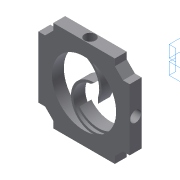
# Autodesk Inventor part: 50_Cube_Insert_Thorlabs
Saved by Autodesk Inventor 2019 (Build 230136000, 136)
## iProperties
Created: 2019-07-01
Part Number: 50_Cube_Insert_Thorlabs
Material: Generic
Document SubType Name: Modeling
Designer: diederichbenedict
Density: 1 g/cm^3
Appearance: Default
Author: diederichbenedict
Autodesk Inventor part; units mm, degrees
ref_plane "YZ Plane" through (0, 0, 0) normal (1, 0, 0) x (0, 1, 0)
ref_plane "Work Plane1" through (0, 0, 10) normal (0, 0, 1) x (1, 0, 0)
sketch "Sketch1" plane through (0, 0, 10) normal (0, 0, 1) x (1, 0, 0)
  line L0 (-4.0299, -0.3538) -> (-2.2322, 1.4439) construction
  arc A0 (-1.4439, 2.2322) -> (-2.2322, 1.4439) centre (-0.9299, 0.9299) ccw construction
  line L1 (-1.4439, 2.2322) -> (0.3538, 4.0299) construction
  line L2 (-37.8299, 42.2137) -> (-37.8299, 45.8299) construction
  line L3 (-37.8299, 45.8299) -> (-4.0299, 45.8299) construction
  line L4 (-4.0299, 45.8299) -> (-4.0299, 42.2137) construction
  line L5 (-4.0299, 4.0299) -> (0.3538, 4.0299) projected
  line L6 (-20.9299, 58.9723) -> (17.1124, 20.9299) construction
  line L7 (17.1124, 20.9299) -> (-20.9299, -17.1124) construction
  line L8 (-20.9299, -17.1124) -> (-58.9723, 20.9299) construction
  line L9 (-58.9723, 20.9299) -> (-20.9299, 58.9723) construction
  line L10 (-20.9299, 58.9723) -> (-20.9299, -17.1124) construction
  line L11 (17.1124, 20.9299) -> (-58.9723, 20.9299) construction
  line L12 (-20.9299, 58.9723) -> (32.8701, 58.9723) construction
  line L13 (-43.4299, 43.4299) -> (1.5701, 43.4299) construction
  line L14 (1.5701, 43.4299) -> (1.5701, -1.5701) construction
  line L15 (1.5701, -1.5701) -> (-43.4299, -1.5701) construction
  line L16 (-43.4299, -1.5701) -> (-43.4299, 43.4299) construction
  line L17 (-43.4299, 43.4299) -> (1.5701, -1.5701) construction
  line L18 (1.5701, 43.4299) -> (-43.4299, -1.5701) construction
  line L19 (-43.4299, 5.3876) -> (-43.4299, 36.4723)
  line L20 (-43.4299, 36.4723) -> (-36.4723, 43.4299)
  line L21 (-36.4723, 43.4299) -> (-5.3876, 43.4299)
  line L22 (-5.3876, 43.4299) -> (1.5701, 36.4723)
  line L23 (1.5701, 36.4723) -> (1.5701, 5.3876)
  line L24 (1.5701, 5.3876) -> (-5.3876, -1.5701)
  line L25 (-5.3876, -1.5701) -> (-36.4723, -1.5701)
  line L26 (-36.4723, -1.5701) -> (-43.4299, 5.3876)
  line L27 (-4.0299, 42.2137) -> (-37.8299, 42.2137) projected
  line L28 (-4.0299, -0.3538) -> (-4.0299, 4.0299) projected
  circle A1 centre (-20.9299, 20.9299) radius 13.3985
  circle A2 centre (-20.9299, 20.9299) radius 15.4895
  point P0 (-37.8299, 4.0299)
  dimension "d18" = 53.8
  dimension "d19" = 45
  dimension "d20" = 53.8
  dimension "d21" = 45
  dimension "d22" = 45
  dimension "d30" = 26.797
  dimension "d36" = 30.979
  constraints: 42 end point, 15 point on line, 4 parallel, 3 midpoint, 3 perpendicular, 2 centre point, 2 coincident, 2 horizontal, 1 equal length
  measures "d18" distance of L6.start L6.end
  measures "d19" angle of L6 L12
  measures "d20" distance of L6.end L7.end
  measures "d21" distance of L14.end L15.end
  measures "d22" distance of L13.end L14.end
  measures "d30" diameter of A1
  measures "d36" diameter of A2
extrude "Extrusion1" add sketch "Sketch1" along normal blind 6.5 contours L28 L24 L25 L26 L19 L20 L27 L22 L23 L5 | L5 L24 L28 | L27 L20 L21 L22 | A1 | A2
ref_plane "Work Plane2" through (-40.9959, 0.8639, 22.2359) normal (0, 0, 1) x (1, 0, 0)
sketch "Sketch3" plane through (0, 0, 10) normal (0, 0, -1) x (-1, 0, 0)
  line L0 (37.8299, -0.4701) -> (37.8299, 4.0299) construction
  line L1 (4.0299, 4.0299) -> (4.0299, -0.4701) construction
  line L2 (37.8299, -0.4701) -> (37.8299, 1.1886) construction
  line L3 (4.0299, -3.9701) -> (4.0299, -0.3538) construction
  line L4 (45.8299, 4.0299) -> (42.2137, 4.0299) construction
  line L5 (-0.3538, 4.0299) -> (-3.9701, 4.0299) construction
  line L6 (-3.9701, 37.8299) -> (-0.3538, 37.8299) construction
  line L7 (4.0299, 42.2137) -> (4.0299, 45.8299) construction
  line L8 (37.8299, 45.8299) -> (37.8299, 42.2137) construction
  line L9 (42.2137, 37.8299) -> (45.8299, 37.8299) construction
  line L10 (37.8299, 37.7299) -> (45.8299, 37.7299)
  line L11 (45.8299, 37.7299) -> (45.8299, 4.1299)
  line L12 (45.8299, 4.1299) -> (37.8299, 4.1299)
  line L13 (37.8299, 4.1299) -> (37.8299, 37.7299)
  line L14 (37.7299, 4.0299) -> (4.1299, 4.0299)
  line L15 (4.1299, 4.0299) -> (4.1299, -3.9701)
  line L16 (4.1299, -3.9701) -> (37.7299, -3.9701)
  line L17 (37.7299, -3.9701) -> (37.7299, 4.0299)
  line L18 (4.0299, 4.1299) -> (-3.9701, 4.1299)
  line L19 (-3.9701, 4.1299) -> (-3.9701, 37.7299)
  line L20 (-3.9701, 37.7299) -> (4.0299, 37.7299)
  line L21 (4.0299, 37.7299) -> (4.0299, 4.1299)
  line L22 (4.1299, 37.8299) -> (37.7299, 37.8299)
  line L23 (37.7299, 37.8299) -> (37.7299, 45.8299)
  line L24 (37.7299, 45.8299) -> (4.1299, 45.8299)
  line L25 (4.1299, 45.8299) -> (4.1299, 37.8299)
  point P0 (0, 0)
  dimension "d23" = 0.1
  dimension "d24" = 0.1
  dimension "d25" = 0.1
  dimension "d26" = 0.1
  dimension "d27" = 0.1
  constraints: 32 end point, 8 parallel, 4 horizontal, 4 perpendicular, 3 point on line
  measures "d23" distance between parallel lines of L8 L23
  measures "d24" distance between parallel lines of L7 L25
  measures "d25" distance between parallel lines of L6 L20
  measures "d26" distance between parallel lines of L5 L18
  measures "d27" distance between parallel lines of L1 L15
extrude "Extrusion3" add sketch "Sketch3" against normal up to surface (6.5 mm away)
sketch "Sketch6" plane through (0, 0, 16.5) normal (0, 0, 1) x (1, 0, 0)
  circle A0 centre (-20.9299, 20.9299) radius 17.5
  circle A1 centre (-20.9299, 20.9299) radius 13.3985
  line L0 (-45.8299, 4.1299) -> (-45.8299, 37.7299) projected
  line L1 (-4.1299, -3.9701) -> (-37.7299, -3.9701) projected
  line L2 (-37.7299, 45.8299) -> (-4.1299, 45.8299) projected
  point P0 (0, 0)
  point P1 (-45.8299, 20.9299)
  point P2 (-20.9299, -3.9701)
  point P3 (-20.9299, 45.8299)
  dimension "d37" = 26.797
  dimension "d38" = 35
  constraints: 3 midpoint, 2 centre point, 2 vertical alignment, 1 coincident, 1 horizontal alignment
  measures "d37" diameter of A1
  measures "d38" diameter of A0
extrude "Extrusion5" cut sketch "Sketch6" against normal blind 12 contours A0 | A1
sketch "Sketch7" plane through (0, 0, 16.5) normal (0, 0, 1) x (1, 0, 0)
  circle A0 centre (-20.9299, 20.9299) radius 17.5 construction
  line L0 (3.9701, 4.1299) -> (0.3124, 4.1299) construction
  line L1 (3.9701, 37.7299) -> (3.9701, 4.1299) construction
  line L2 (0.3124, 37.7299) -> (3.9701, 37.7299) construction
  line L3 (0.3124, 37.7299) -> (-4.1299, 42.1723) construction
  line L4 (-4.1299, 45.8299) -> (-4.1299, 42.1723) construction
  line L5 (-37.7299, 45.8299) -> (-4.1299, 45.8299) construction
  line L6 (-37.7299, 42.1723) -> (-37.7299, 45.8299) construction
  line L7 (-37.7299, 42.1723) -> (-42.1723, 37.7299) construction
  line L8 (-45.8299, 37.7299) -> (-42.1723, 37.7299) construction
  line L9 (-45.8299, 4.1299) -> (-45.8299, 37.7299) construction
  line L10 (-42.1723, 4.1299) -> (-45.8299, 4.1299) construction
  line L11 (-42.1723, 4.1299) -> (-37.7299, -0.3124) construction
  line L12 (-37.7299, -3.9701) -> (-37.7299, -0.3124) construction
  line L13 (-4.1299, -3.9701) -> (-37.7299, -3.9701) construction
  line L14 (-4.1299, -0.3124) -> (-4.1299, -3.9701) construction
  line L15 (-4.1299, -0.3124) -> (0.3124, 4.1299) construction
  circle A1 centre (-20.9299, 20.9299) radius 17.5 construction
  line L16 (-5.7745, 12.1799) -> (-36.0854, 12.1799) construction
  line L17 (-36.0854, 12.1799) -> (-20.9299, 38.4299) construction
  line L18 (-20.9299, 38.4299) -> (-5.7745, 12.1799) construction
  circle A2 centre (-22.4299, 22.4299) radius 7 construction
  arc A3 (-20.9299, 38.4299) -> (-24.2565, 38.1108) centre (-20.9299, 20.9299) ccw
  line L19 (-28.4921, 18.9299) -> (-22.4299, 29.4299)
  line L20 (-22.4299, 29.4299) -> (-16.3678, 18.9299)
  line L21 (-16.3678, 18.9299) -> (-28.4921, 18.9299)
  arc A4 (-20.9299, 38.4299) -> (-28.4921, 18.9299) centre (-15.4327, 25.0818) ccw
  arc A5 (-24.2565, 38.1108) -> (-29.7634, 18.5819) centre (-15.4327, 25.0818) ccw
  line L22 (-29.7634, 18.5819) -> (-28.4921, 18.9299)
  arc A6 (-5.7745, 12.1799) -> (-22.4299, 29.4299) centre (-24.2867, 10.9714) ccw
  arc A7 (-5.7745, 12.1799) -> (-4.7215, 14.3316) centre (-20.9299, 20.9299) ccw
  arc A8 (-4.7215, 14.3316) -> (-22.0384, 30.6954) centre (-24.2867, 10.9714) ccw
  line L23 (-22.0384, 30.6954) -> (-22.4299, 29.4299)
  arc A9 (-36.0854, 12.1799) -> (-16.3678, 18.9299) centre (-30.247, 27.2992) ccw
  arc A10 (-36.0854, 12.1799) -> (-34.9298, 10.4297) centre (-20.9299, 20.9299) ccw
  arc A11 (-34.9298, 10.4297) -> (-15.0056, 18.6848) centre (-30.247, 27.2992) ccw
  line L24 (-15.0056, 18.6848) -> (-16.3678, 18.9299)
  dimension "d93" = 14
  dimension "d94" = 1.5
  dimension "d95" = 1.5
  dimension "d96" = 1.3
  dimension "d97" = 1.3
  dimension "d98" = 1.3
  constraints: 22 point on circle, 18 end point, 9 centre point, 5 concentric, 2 coincident, 2 parallel, 17 other
  measures "d94" horizontal distance of A0.centre point (-22.43, 22.43)
  measures "d95" horizontal distance of A0.centre point (-22.43, 22.43)
  measures "d96" radial gap between concentric circles of A5 A4
  measures "d97" radial gap between concentric circles of A6 A8
  measures "d98" radial gap between concentric circles of A11 A9
extrude "Extrusion6" add sketch "Sketch7" against normal up to surface (6.5 mm away) contours A4 L22 A5 A3 | L23 A8 A7 A6 | L24 A11 A10 A9
sketch "Sketch8" plane through (-37.7299, 45.8299, 10) normal (0, 1, 0) x (1, 0, 0)
  line L0 (0, 0) -> (33.6, 0) projected
  line L1 (0, -6.5) -> (33.6, -6.5) projected
  line L2 (33.6, 0) -> (33.6, -6.5) projected
  line L3 (0, 0) -> (0, -6.5) projected
  point P0 (37.7299, 10)
  point P1 (16.8, -3.25)
  point P2 (16.8, 0)
  point P3 (16.8, -6.5)
  point P4 (33.6, -3.25)
  point P5 (0, -3.25)
  constraints: 4 midpoint, 2 horizontal alignment, 2 vertical alignment
hole "Hole1" at (-20.9299, 45.8299, 13.25) direction (0, -1, 0) diameter 2.9 depth 11 tip angle 118 counterbore diameter 6 counterbore depth 6
sketch "Sketch9" plane through (3.9701, 4.1299, 10) normal (1, 0, 0) x (0, 0, -1)
  line L0 (0, 0) -> (0, 33.6) projected
  line L1 (-6.5, 33.6) -> (-6.5, 0) projected
  line L2 (0, 33.6) -> (-6.5, 33.6) projected
  line L3 (0, 0) -> (-6.5, 0) projected
  point P0 (10, -4.1299)
  point P1 (-3.25, 16.8)
  point P2 (0, 16.8)
  point P3 (-6.5, 16.8)
  point P4 (-3.25, 33.6)
  point P5 (-3.25, 0)
  constraints: 4 midpoint, 2 horizontal alignment, 2 vertical alignment
hole "Hole2" at (3.9701, 20.9299, 13.25) direction (-1, 0, 0) diameter 2.9 depth 11 tip angle 118 counterbore diameter 6 counterbore depth 6
body "Solid1"
